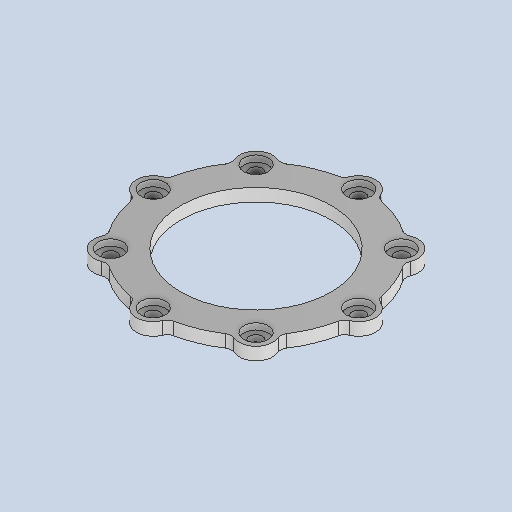
# Autodesk Inventor part: Outer_flange
Saved by Autodesk Inventor 2022.4 (Build 264492000, 492)
## iProperties
Created: 2021-09-26
Part Number: Outer_flange
Material: アルミニウム 2014-T4
Document SubType Name: Modeling
Designer: Masato Kubotera
Density: 2.8 g/cm^3
Appearance: 滑らか - 淡い灰色
Mass: 8.65051 g
Surface Area: 34.3389 cm^2
Volume: 3.08947 cm^3
Description: A2017 T3
Author: Masato Kubotera
Keywords: A2017 T4
Autodesk Inventor part; units mm, degrees
ref_plane "YZ Plane" through (0, 0, 0) normal (1, 0, 0) x (0, 1, 0)
ref_plane "XZ Plane" through (0, 0, 0) normal (0, 1, 0) x (-1, 0, 0)
ref_plane "XY Plane" through (0, 0, 0) normal (0, 0, 1) x (1, 0, 0)
derived "Outer_support_stand.ipt"
sketch "スケッチ1" plane through (0, 0, 0) normal (0, 0, 1) x (1, 0, 0)
  line L0 (-62, 30.75) -> (62, 30.75)
  line L1 (62, -30.75) -> (-62, -30.75)
  line L2 (-62, 30.75) -> (62, -30.75) construction
  line L3 (62, 30.75) -> (-62, -30.75) construction
  line L4 (0, 30.75) -> (0, -30.75) construction
  circle A0 centre (-44, 2.25) radius 10.5 construction
  line L5 (-57.5, 1.25) -> (-30.5, 1.25) construction
  line L6 (-30.5, 1.25) -> (-30.5, -25.75) construction
  line L7 (-30.5, -25.75) -> (-57.5, -25.75) construction
  line L8 (-57.5, -25.75) -> (-57.5, 1.25) construction
  line L9 (-44, 1.25) -> (-44, -25.75) construction
  line L10 (-57.5, -12.25) -> (-30.5, -12.25) construction
  circle A1 centre (-57.5, 1.25) radius 1.5
  circle A2 centre (-57.5, -25.75) radius 1.5
  circle A3 centre (-30.5, 1.25) radius 1.5
  circle A4 centre (-30.5, -25.75) radius 1.5
  line L11 (-27.5, 14.75) -> (-22.5, 14.75) construction
  line L12 (-22.5, 14.75) -> (-22.5, -10.25) construction
  line L13 (-22.5, -10.25) -> (-27.5, -10.25) construction
  line L14 (-27.5, -10.25) -> (-27.5, 14.75) construction
  line L15 (-27.5, 14.75) -> (-22.5, -10.25) construction
  line L16 (-22.5, 14.75) -> (-27.5, -10.25) construction
  line L17 (-27.55, 14.8) -> (-22.45, 14.8)
  line L18 (-22.45, 14.8) -> (-22.45, -10.3)
  line L19 (-22.45, -10.3) -> (-27.55, -10.3)
  line L20 (-27.55, -10.3) -> (-27.55, 14.8)
  line L21 (-27.55, 14.8) -> (-22.45, -10.3) construction
  line L22 (-22.45, 14.8) -> (-27.55, -10.3) construction
  line L23 (-27.55, 2.25) -> (-22.45, 2.25) construction
  line L24 (-25, 14.8) -> (-25, -10.3) construction
  arc A5 (-27.55, 14.8) -> (-27.55, 12.7) centre (-27.55, 13.75) ccw
  arc A6 (-22.45, 12.7) -> (-22.45, 14.8) centre (-22.45, 13.75) ccw
  arc A7 (-27.55, -8.2) -> (-27.55, -10.3) centre (-27.55, -9.25) ccw
  arc A8 (-22.45, -10.3) -> (-22.45, -8.2) centre (-22.45, -9.25) ccw
  circle A9 centre (-25, 27.75) radius 1.55
  line L25 (-22.5, -17.25) -> (-27.5, -17.25) construction
  circle A10 centre (-25, -23.25) radius 1.55
  circle A11 centre (-44, 2.25) radius 11
  line L26 (62, 2.25) -> (-62, 2.25) construction
  line L27 (-60, 14.25) -> (-28, 14.25) construction
  line L28 (-28, 14.25) -> (-28, -28.75) construction
  line L29 (-28, -28.75) -> (-60, -28.75) construction
  line L30 (-60, -28.75) -> (-60, 14.25) construction
  line L31 (-60, 14.25) -> (-28, -28.75) construction
  line L32 (-28, 14.25) -> (-60, -28.75) construction
  line L33 (-62, 30.75) -> (-62, -30.75) construction
  line L34 (62, 30.75) -> (62, -30.75) construction
  circle A12 centre (-44, 2.25) radius 12.5 construction
  circle A13 centre (-44, 2.25) radius 20.5 construction
  circle A14 centre (-44, 2.25) radius 28.5 construction
  circle A15 centre (-44, 26.75) radius 1.25 construction
  circle A16 centre (-61.3241, 19.5741) radius 1.25 construction
  circle A17 centre (-68.5, 2.25) radius 1.25 construction
  circle A18 centre (-61.3241, -15.0741) radius 1.25 construction
  circle A19 centre (-44, -22.25) radius 1.25 construction
  circle A20 centre (-26.6759, -15.0741) radius 1.25 construction
  circle A21 centre (-19.5, 2.25) radius 1.25 construction
  circle A22 centre (-26.6759, 19.5741) radius 1.25 construction
  line L35 (-62, -21.122) -> (-62, -30.75)
  circle A23 centre (57.5, 1.25) radius 1.5
  circle A24 centre (57.5, -25.75) radius 1.5
  circle A25 centre (30.5, 1.25) radius 1.5
  circle A26 centre (30.5, -25.75) radius 1.5
  line L36 (27.55, 14.8) -> (22.45, 14.8)
  line L37 (22.45, 14.8) -> (22.45, -10.3)
  line L38 (22.45, -10.3) -> (27.55, -10.3)
  line L39 (27.55, -10.3) -> (27.55, 14.8)
  arc A27 (27.55, 12.7) -> (27.55, 14.8) centre (27.55, 13.75) ccw
  arc A28 (22.45, 14.8) -> (22.45, 12.7) centre (22.45, 13.75) ccw
  arc A29 (22.45, -8.2) -> (22.45, -10.3) centre (22.45, -9.25) ccw
  arc A30 (27.55, -10.3) -> (27.55, -8.2) centre (27.55, -9.25) ccw
  circle A31 centre (25, 27.75) radius 1.55
  circle A32 centre (25, -23.25) radius 1.55
  circle A33 centre (44, 2.25) radius 11
  circle A34 centre (44, 26.75) radius 1.25
  circle A35 centre (61.3241, 19.5741) radius 1.25
  circle A36 centre (68.5, 2.25) radius 1.25
  circle A37 centre (61.3241, -15.0741) radius 1.25
  circle A38 centre (44, -22.25) radius 1.25
  circle A39 centre (26.6759, -15.0741) radius 1.25
  circle A40 centre (19.5, 2.25) radius 1.25
  circle A41 centre (26.6759, 19.5741) radius 1.25
  line L40 (62, -21.122) -> (62, -30.75)
  circle A42 centre (-44, 2.25) radius 20.51
  circle A43 centre (-44, 2.25) radius 18.5
  circle A44 centre (-44, 2.25) radius 28.5
  circle A45 centre (-44, 26.75) radius 1.55
  circle A46 centre (-61.3241, 19.5741) radius 1.55
  circle A47 centre (-68.5, 2.25) radius 1.55
  circle A48 centre (-61.3241, -15.0741) radius 1.55
  circle A49 centre (-44, -22.25) radius 1.55
  circle A50 centre (-26.6759, -15.0741) radius 1.55
  circle A51 centre (-19.5, 2.25) radius 1.55
  circle A52 centre (-26.6759, 19.5741) radius 1.55
  line L41 (-68.5, 2.25) -> (-73.5, 2.25) construction
  circle A53 centre (-26.6759, -15.0741) radius 6.25 construction
  circle A54 centre (-44, 2.25) radius 24.5 construction
  circle A55 centre (-44, 26.75) radius 3.05
  circle A56 centre (-61.3241, 19.5741) radius 3.05
  circle A57 centre (-68.5, 2.25) radius 3.05
  circle A58 centre (-44, -22.25) radius 3.05
  circle A59 centre (-26.6759, -15.0741) radius 3.05
  circle A60 centre (-19.5, 2.25) radius 3.05
  circle A61 centre (-26.6759, 19.5741) radius 3.05
  circle A62 centre (-61.3241, -15.0741) radius 3.05
  circle A63 centre (-44, 2.25) radius 17.9
  circle A64 centre (-44, 26.75) radius 2.9
  circle A65 centre (-61.3241, 19.5741) radius 2.9
  circle A66 centre (-68.5, 2.25) radius 2.9
  circle A67 centre (-61.3241, -15.0741) radius 2.9
  circle A68 centre (-44, -22.25) radius 2.9
  circle A69 centre (-26.6759, -15.0741) radius 2.9
  circle A70 centre (-19.5, 2.25) radius 2.9
  circle A71 centre (-26.6759, 19.5741) radius 2.9
  circle A72 centre (-30.5, -25.75) radius 2.4
  arc A73 (-44, 30.75) -> (-47.969, 27.2469) centre (-44, 26.75) ccw
  arc A74 (-58.8689, 22.732) -> (-64.1525, 22.4025) centre (-61.3241, 19.5741) ccw
  arc A75 (-47.969, 27.2469) -> (-58.8689, 22.732) centre (-44, 2.25) ccw
  arc A76 (-64.1525, 22.4025) -> (-64.482, 17.1189) centre (-61.3241, 19.5741) ccw
  arc A77 (-64.482, 17.1189) -> (-68.9969, 6.219) centre (-44, 2.25) ccw
  arc A78 (-68.9969, 6.219) -> (-72.5, 2.25) centre (-68.5, 2.25) ccw
  arc A79 (-72.5, 2.25) -> (-68.9969, -1.719) centre (-68.5, 2.25) ccw
  arc A80 (-68.9969, -1.719) -> (-64.482, -12.6189) centre (-44, 2.25) ccw
  arc A81 (-64.482, -12.6189) -> (-64.1525, -17.9025) centre (-61.3241, -15.0741) ccw
  arc A82 (-64.1525, -17.9025) -> (-58.8689, -18.232) centre (-61.3241, -15.0741) ccw
  arc A83 (-58.8689, -18.232) -> (-47.969, -22.7469) centre (-44, 2.25) ccw
  arc A84 (-47.969, -22.7469) -> (-44, -26.25) centre (-44, -22.25) ccw
  arc A85 (-44, -26.25) -> (-40.031, -22.7469) centre (-44, -22.25) ccw
  arc A86 (-40.031, -22.7469) -> (-29.1311, -18.232) centre (-44, 2.25) ccw
  arc A87 (-29.1311, -18.232) -> (-23.8475, -17.9025) centre (-26.6759, -15.0741) ccw
  arc A88 (-23.8475, -17.9025) -> (-23.518, -12.6189) centre (-26.6759, -15.0741) ccw
  arc A89 (-23.518, -12.6189) -> (-19.0031, -1.719) centre (-44, 2.25) ccw
  arc A90 (-19.0031, -1.719) -> (-15.5, 2.25) centre (-19.5, 2.25) ccw
  arc A91 (-15.5, 2.25) -> (-19.0031, 6.219) centre (-19.5, 2.25) ccw
  arc A92 (-19.0031, 6.219) -> (-23.518, 17.1189) centre (-44, 2.25) ccw
  arc A93 (-23.518, 17.1189) -> (-23.8475, 22.4025) centre (-26.6759, 19.5741) ccw
  arc A94 (-23.8475, 22.4025) -> (-29.1311, 22.732) centre (-26.6759, 19.5741) ccw
  arc A95 (-29.1311, 22.732) -> (-40.031, 27.2469) centre (-44, 2.25) ccw
  arc A96 (-40.031, 27.2469) -> (-44, 30.75) centre (-44, 26.75) ccw
  arc A97 (-47.969, 27.2469) -> (-58.8689, 22.732) centre (-44, 2.25) ccw
  arc A98 (-44, 30.75) -> (-47.969, 27.2469) centre (-44, 26.75) ccw
  arc A99 (-58.8689, 22.732) -> (-64.482, 17.1189) centre (-61.3241, 19.5741) ccw
  arc A100 (-64.482, 17.1189) -> (-68.9969, 6.219) centre (-44, 2.25) ccw
  arc A101 (-68.9969, 6.219) -> (-68.9969, -1.719) centre (-68.5, 2.25) ccw
  arc A102 (-68.9969, -1.719) -> (-64.482, -12.6189) centre (-44, 2.25) ccw
  arc A103 (-64.482, -12.6189) -> (-62, -19.0166) centre (-61.3241, -15.0741) ccw
  line L42 (-62, -19.0166) -> (-62, -21.122)
  arc A104 (58.8689, 22.732) -> (47.969, 27.2469) centre (44, 2.25) ccw
  arc A105 (47.969, 27.2469) -> (44, 30.75) centre (44, 26.75) ccw
  arc A106 (64.482, 17.1189) -> (58.8689, 22.732) centre (61.3241, 19.5741) ccw
  arc A107 (68.9969, 6.219) -> (64.482, 17.1189) centre (44, 2.25) ccw
  arc A108 (68.9969, -1.719) -> (68.9969, 6.219) centre (68.5, 2.25) ccw
  arc A109 (64.482, -12.6189) -> (68.9969, -1.719) centre (44, 2.25) ccw
  arc A110 (62, -19.0166) -> (64.482, -12.6189) centre (61.3241, -15.0741) ccw
  line L43 (62, -19.0166) -> (62, -21.122)
  line L44 (19.5, 25.75) -> (-19.5, 25.75)
  line L45 (-19.5, 25.75) -> (-19.5, 7.25)
  circle A111 centre (-25, 27.75) radius 2.75 construction
  line L46 (-15.1699, 4.75) -> (15.1699, 4.75)
  arc A112 (-15.1699, 4.75) -> (-19.5, 7.25) centre (-19.5, 2.25) ccw
  line L47 (19.5, 25.75) -> (19.5, 7.25)
  arc A113 (19.5, 7.25) -> (15.1699, 4.75) centre (19.5, 2.25) ccw
  line L48 (-15.1699, -0.25) -> (15.1699, -0.25)
  arc A114 (-19.5, -2.75) -> (-15.1699, -0.25) centre (-19.5, 2.25) ccw
  arc A115 (15.1699, -0.25) -> (19.5, -2.75) centre (19.5, 2.25) ccw
  line L49 (-19.5, -2.75) -> (-19.5, -25.75)
  line L50 (-19.5, -25.75) -> (19.5, -25.75)
  line L51 (19.5, -25.75) -> (19.5, -2.75)
  point P0 (0, 0)
  point P1 (-25, 2.25)
  point P2 (-44, -7.25)
  point P3 (-23.8475, 22.4025)
  point P4 (-64.1525, -17.9025)
  point P5 (-44, -26.25)
  point P6 (-23.8475, -17.9025)
  point P7 (-15.5, 2.25)
  point P8 (-25, 2.25)
  point P9 (-23.326, 21.76)
  point P10 (-23.2248, 21.76)
  point P11 (-23.8475, 22.4025)
  point P12 (-64.1525, -17.9025)
  point P13 (-44, -26.25)
  point P14 (-23.8475, -17.9025)
  point P15 (-15.5, 2.25)
  point P16 (-23.8475, 22.4025)
  point P17 (27.9147, 19.7411)
  point P18 (27.51, 18.6431)
  point P19 (27.55, -8.2)
  point P20 (-27.51, 18.6431)
  point P21 (-27.9147, 19.7411)
  point P22 (-26.4271, 21.76)
  point P23 (-26.9247, 21.76)
  point P24 (-27.51, 20.5051)
  point P25 (27.51, 20.5051)
  point P26 (26.9247, 21.76)
  point P27 (26.4271, 21.76)
  point P28 (-47, 30.75)
  point P29 (47, 30.75)
  dimension "d1" = 35.8
  dimension "d7" = 5.8
  dimension "d8" = 5.8
  dimension "d9" = 5.8
  dimension "d10" = 5.8
  dimension "d11" = 5.8
  dimension "d12" = 5.8
  dimension "d13" = 5.8
  dimension "d14" = 5.8
  measures "d1" diameter of A63
  measures "d7" diameter of A64
  measures "d8" diameter of A65
  measures "d9" diameter of A66
  measures "d10" diameter of A67
  measures "d11" diameter of A68
  measures "d12" diameter of A69
  measures "d13" diameter of A70
  measures "d14" diameter of A71
extrude "押し出し1" add sketch "スケッチ1" along normal blind 3 contours A96 A95 A94 A93 A92 A6 L17 A5 A42 A7 L19 A8 A89 A88 A87 A86 A85 A84 A83 A82 A81 A80 A79 A78 A77 A76 A74 A75 A73 | L45 A112 A92 A91 A90 A89 A114 L49 A8 L18 A60 A6 | A92 A112 L45 | A92 A6 L18 | L18 A60 L19 L20 A42 L17 | L20 A42 A5 | A89 L49 A114 | A60 L18 | L18 A60 | A42 L20 A43 | L20 A5 A42 | A5 L20 A43 A7 A42 | A42 L20 A7 | A7 L20 A42 | A89 A8 L18 | A43 L20 A63 | L20 A63 A43 | A55 | A56 | A57 | A58 | A59 | A61 | A62
extrude "押し出し2" add sketch "スケッチ1" along normal blind 1.5 contours A64 | A65 | A66 | A67 | A68 | A69 | A70 | A71
fillet "フィレット1" radius 2 16 edges at (-58.8689, 22.732, 1.5) (-40.031, 27.2469, 1.5) (-47.969, 27.2469, 1.5) (-29.1311, 22.732, 1.5) (-23.518, 17.1189, 1.5) (-19.0031, -1.719, 1.5) (-23.518, -12.6189, 1.5) (-40.031, -22.7469, 1.5) (-19.0031, 6.219, 1.5) (-64.482, 17.1189, 1.5) (-68.9969, 6.219, 1.5) (-68.9969, -1.719, 1.5) (-64.482, -12.6189, 1.5) (-58.8689, -18.232, 1.5) (-47.969, -22.7469, 1.5) (-29.1311, -18.232, 1.5)
equation "\"d8\" = d7"
equation "\"d9\" = d7"
equation "\"d10\" = d7"
equation "\"d11\" = d7"
equation "\"d12\" = d7"
equation "\"d13\" = d7"
equation "\"d14\" = d7"
